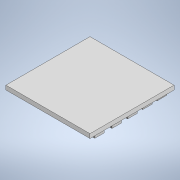
# Autodesk Inventor part: hall_toll
Saved by Autodesk Inventor 2021 (Build 250183000, 183)
## iProperties
Created: 2021-03-01
Part Number: hall_toll
Material: Generic
Document SubType Name: Modeling
Designer: Patrick
Density: 1 g/cm^3
Appearance: Default
Author: Patrick
Autodesk Inventor part; units mm, degrees
(part 1 of 2)
ref_plane "YZ Plane" through (0, 0, 0) normal (1, 0, 0) x (0, 1, 0)
ref_plane "XZ Plane" through (0, 0, 0) normal (0, 1, 0) x (-1, 0, 0)
ref_plane "XY Plane" through (0, 0, 0) normal (0, 0, 1) x (1, 0, 0)
sketch "Sketch1" plane through (0, 0, 0) normal (0, 1, 0) x (-1, 0, 0)
  line L0 (0, -5.8586) -> (50.8, -5.8586)
  line L1 (50.8, -5.8586) -> (50.8, -56.6586)
  line L2 (50.8, -56.6586) -> (0, -56.6586)
  line L3 (0, -56.6586) -> (0, -5.8586)
  line L4 (0, 0) -> (0, 2.7804) construction
  line L5 (15.8266, -10.75) -> (12.7532, -10.75)
  line L6 (12.7532, -10.75) -> (12.7532, -14.7378)
  line L7 (12.7532, -14.7378) -> (15.8266, -14.7378)
  line L8 (15.8266, -14.7378) -> (15.8266, -10.75)
  line L9 (15.8266, -10.75) -> (12.7532, -14.7378) construction
  line L10 (12.7532, -10.75) -> (15.8266, -14.7378) construction
  line L11 (16.6394, -9.9372) -> (11.9404, -9.9372)
  line L12 (11.9404, -9.9372) -> (11.9404, -15.5506)
  line L13 (11.9404, -15.5506) -> (16.6394, -15.5506)
  line L14 (16.6394, -15.5506) -> (16.6394, -9.9372)
  line L15 (16.6394, -9.9372) -> (11.9404, -15.5506) construction
  line L16 (11.9404, -9.9372) -> (16.6394, -15.5506) construction
  line L17 (11.9404, -10.9532) -> (16.6394, -10.9532)
  line L18 (16.6394, -10.9532) -> (16.6394, -14.5346)
  line L19 (16.6394, -14.5346) -> (11.9404, -14.5346)
  line L20 (11.9404, -14.5346) -> (11.9404, -10.9532)
  line L21 (11.9404, -10.9532) -> (16.6394, -14.5346) construction
  line L22 (16.6394, -10.9532) -> (11.9404, -14.5346) construction
  line L23 (15.8118, -21.1328) -> (12.6884, -21.1328)
  line L24 (12.6884, -21.1328) -> (12.6884, -25.1706)
  line L25 (12.6884, -25.1706) -> (15.8118, -25.1706)
  line L26 (15.8118, -25.1706) -> (15.8118, -21.1328)
  line L27 (15.8118, -21.1328) -> (12.6884, -25.1706) construction
  line L28 (12.6884, -21.1328) -> (15.8118, -25.1706) construction
  line L29 (16.6246, -20.32) -> (11.8756, -20.32)
  line L30 (11.8756, -20.32) -> (11.8756, -25.9834)
  line L31 (11.8756, -25.9834) -> (16.6246, -25.9834)
  line L32 (16.6246, -25.9834) -> (16.6246, -20.32)
  line L33 (16.6246, -20.32) -> (11.8756, -25.9834) construction
  line L34 (11.8756, -20.32) -> (16.6246, -25.9834) construction
  line L35 (11.8756, -21.361) -> (16.6246, -21.361)
  line L36 (16.6246, -21.361) -> (16.6246, -24.9424)
  line L37 (16.6246, -24.9424) -> (11.8756, -24.9424)
  line L38 (11.8756, -24.9424) -> (11.8756, -21.361)
  line L39 (11.8756, -21.361) -> (16.6246, -24.9424) construction
  line L40 (16.6246, -21.361) -> (11.8756, -24.9424) construction
  line L41 (12.6374, -34.9027) -> (15.8108, -34.9027)
  line L42 (11.8246, -34.6495) -> (11.8246, -31.0681)
  line L43 (16.6236, -34.6495) -> (11.8246, -34.6495)
  line L44 (11.8246, -35.7155) -> (16.6236, -35.7155)
  line L45 (12.6374, -30.8149) -> (12.6374, -34.9027)
  line L46 (11.8246, -30.0021) -> (11.8246, -35.7155)
  line L47 (15.8108, -30.8149) -> (12.6374, -34.9027) construction
  line L48 (15.8108, -34.9027) -> (15.8108, -30.8149)
  line L49 (12.6374, -30.8149) -> (15.8108, -34.9027) construction
  line L50 (16.6236, -31.0681) -> (11.8246, -34.6495) construction
  line L51 (16.6236, -31.0681) -> (16.6236, -34.6495)
  line L52 (11.8246, -31.0681) -> (16.6236, -34.6495) construction
  line L53 (11.8246, -30.0021) -> (16.6236, -35.7155) construction
  line L54 (16.6236, -30.0021) -> (11.8246, -35.7155) construction
  line L55 (16.6236, -35.7155) -> (16.6236, -30.0021)
  line L56 (11.8246, -31.0681) -> (16.6236, -31.0681)
  line L57 (16.6236, -30.0021) -> (11.8246, -30.0021)
  line L58 (15.8108, -30.8149) -> (12.6374, -30.8149)
  line L59 (15.8942, -40.2355) -> (12.6708, -40.2355)
  line L60 (12.6708, -44.3733) -> (15.8942, -44.3733)
  line L61 (16.707, -40.5137) -> (16.707, -44.0951)
  line L62 (11.858, -44.0951) -> (11.858, -40.5137)
  line L63 (12.6708, -40.2355) -> (12.6708, -44.3733)
  line L64 (15.8942, -44.3733) -> (15.8942, -40.2355)
  line L65 (11.858, -40.5137) -> (16.707, -40.5137)
  line L66 (16.707, -44.0951) -> (11.858, -44.0951)
  line L67 (15.8942, -40.2355) -> (12.6708, -44.3733) construction
  line L68 (12.6708, -40.2355) -> (15.8942, -44.3733) construction
  line L69 (16.707, -39.4227) -> (11.858, -39.4227)
  line L70 (11.858, -45.1861) -> (16.707, -45.1861)
  line L71 (16.707, -40.5137) -> (11.858, -44.0951) construction
  line L72 (11.858, -40.5137) -> (16.707, -44.0951) construction
  line L73 (16.707, -45.1861) -> (16.707, -39.4227)
  line L74 (11.858, -39.4227) -> (16.707, -45.1861) construction
  line L75 (16.707, -39.4227) -> (11.858, -45.1861) construction
  line L76 (11.858, -39.4227) -> (11.858, -45.1861)
  line L77 (12.6807, -53.397) -> (15.9541, -53.397)
  line L78 (11.8679, -53.0938) -> (11.8679, -49.5124)
  line L79 (12.6807, -49.2092) -> (12.6807, -53.397)
  line L80 (16.7669, -53.0938) -> (11.8679, -53.0938)
  line L81 (11.8679, -54.2098) -> (16.7669, -54.2098)
  line L82 (15.9541, -49.2092) -> (12.6807, -53.397) construction
  line L83 (15.9541, -53.397) -> (15.9541, -49.2092)
  line L84 (15.9541, -49.2092) -> (12.6807, -49.2092)
  line L85 (16.7669, -49.5124) -> (16.7669, -53.0938)
  line L86 (11.8679, -48.3964) -> (11.8679, -54.2098)
  line L87 (16.7669, -49.5124) -> (11.8679, -53.0938) construction
  line L88 (11.8679, -49.5124) -> (16.7669, -53.0938) construction
  line L89 (11.8679, -49.5124) -> (16.7669, -49.5124)
  line L90 (16.7669, -48.3964) -> (11.8679, -48.3964)
  line L91 (16.7669, -48.3964) -> (11.8679, -54.2098) construction
  line L92 (11.8679, -48.3964) -> (16.7669, -54.2098) construction
  line L93 (16.7669, -54.2098) -> (16.7669, -48.3964)
  line L94 (12.6807, -49.2092) -> (15.9541, -53.397) construction
  point P0 (14.2899, -12.7439)
  point P1 (14.2899, -12.7439)
  point P2 (14.2899, -12.7439)
  point P3 (14.2899, -12.7439)
  point P4 (14.2899, -12.7439)
  point P5 (14.2501, -23.1517)
  point P6 (14.2501, -23.1517)
  point P7 (14.2501, -23.1517)
  point P8 (14.2501, -23.1517)
  point P9 (14.2501, -23.1517)
  point P10 (14.2241, -32.8588)
  point P11 (14.2241, -32.8588)
  point P12 (14.2241, -32.8588)
  point P13 (14.2241, -32.8588)
  point P14 (14.2241, -32.8588)
  point P15 (14.2825, -42.3044)
  point P16 (14.2825, -42.3044)
  point P17 (14.2825, -42.3044)
  point P18 (14.2825, -42.3044)
  point P19 (14.2825, -42.3044)
  point P20 (14.3174, -51.3031)
  point P21 (14.3174, -51.3031)
  point P22 (14.3174, -51.3031)
  point P23 (14.3174, -51.3031)
  point P24 (14.3174, -51.3031)
  point P25 (12.6807, -53.0938)
  point P26 (12.6807, -49.5124)
  point P27 (12.6708, -44.0951)
  point P28 (12.6708, -40.5137)
  point P29 (12.6374, -34.6495)
  point P30 (12.6374, -31.0681)
  point P31 (12.6884, -21.361)
  point P32 (12.6884, -24.9424)
  point P33 (12.7532, -14.5346)
  point P34 (12.7532, -10.9532)
  dimension "d1" = 50.8
  dimension "d8" = 3.9878
  dimension "d9" = 3.0734
  dimension "d10" = 0.8128
  dimension "d11" = 0.8128
  dimension "d12" = 3.5814
  dimension "d13" = 4.0378
  dimension "d14" = 3.1234
  dimension "d15" = 0.8128
  dimension "d16" = 0.8128
  dimension "d17" = 3.5814
  dimension "d18" = 4.0878
  dimension "d19" = 3.1734
  dimension "d20" = 0.8128
  dimension "d21" = 0.8128
  dimension "d22" = 3.5814
  dimension "d23" = 4.1378
  dimension "d24" = 3.2234
  dimension "d25" = 0.8128
  dimension "d26" = 0.8128
  dimension "d27" = 3.5814
  dimension "d28" = 4.1878
  dimension "d29" = 3.2734
  dimension "d30" = 0.8128
  dimension "d31" = 0.8128
  dimension "d32" = 3.5814
  constraints: 190 end point, 50 midpoint, 32 parallel, 16 horizontal, 16 perpendicular, 5 collinear, 1 vertical
  measures "d1" distance between parallel lines of L3 L1
  measures "d8" distance of L5.end L6.end
  measures "d9" distance between parallel lines of L6 L8
  measures "d10" distance between parallel lines of L13 L7
  measures "d11" distance between parallel lines of L12 L6
  measures "d12" distance between parallel lines of L19 L17
  measures "d13" distance of L24.start L25.start
  measures "d14" distance between parallel lines of L24 L26
  measures "d15" distance between parallel lines of L31 L25
  measures "d16" distance between parallel lines of L30 L24
  measures "d17" distance between parallel lines of L37 L35
  measures "d18" distance of L58.end L41.start
  measures "d19" distance between parallel lines of L45 L48
  measures "d20" distance between parallel lines of L44 L41
  measures "d21" distance between parallel lines of L46 L45
  measures "d22" distance between parallel lines of L43 L56
  measures "d23" distance of L63.start L60.start
  measures "d24" distance between parallel lines of L63 L64
  measures "d25" distance between parallel lines of L70 L60
  measures "d26" distance between parallel lines of L76 L63
  measures "d27" distance between parallel lines of L66 L65
  measures "d28" distance of L84.end L79.end
  measures "d29" distance between parallel lines of L79 L83
  measures "d30" distance between parallel lines of L81 L77
  measures "d31" distance between parallel lines of L86 L79
  measures "d32" distance between parallel lines of L80 L89
extrude "Extrusion2" add sketch "Sketch1" along normal blind 2.54 contours L0 L1 L2 L3 | L8 L17 L6 L5 | L5 L6 L17 L12 L11 L14 L8 | L17 L14 L19 L8 | L8 L19 L6 L17 | L6 L19 L12 L17 | L19 L14 L13 L12 L6 L7 L8 | L8 L7 L6 L19 | L26 L35 L24 L23 | L23 L24 L35 L30 L29 L32 L26 | L35 L32 L37 L26 | L26 L37 L24 L35 | L24 L37 L30 L35 | L37 L32 L31 L30 L24 L25 L26 | L26 L25 L24 L37 | L45 L43 L48 L41 | L41 L48 L43 L55 L44 L46 L45 | L45 L56 L48 L43 | L43 L42 L56 L45 | L48 L56 L51 L43 | L56 L46 L57 L55 L48 L58 L45 | L45 L58 L48 L56 | L64 L65 L63 L59 | L59 L63 L65 L76 L69 L73 L64 | L65 L61 L66 L64 | L64 L66 L63 L65 | L63 L66 L62 L65 | L66 L73 L70 L76 L63 L60 L64 | L64 L60 L63 L66 | L79 L80 L83 L77 | L77 L83 L80 L93 L81 L86 L79 | L80 L78 L89 L79 | L79 L89 L83 L80 | L83 L89 L85 L80 | L89 L86 L90 L93 L83 L84 L79 | L79 L84 L83 L89
sketch "Sketch2" plane through (0, 0, 0) normal (0, -1, 0) x (1, 0, 0)
  line L0 (0, -5.8586) -> (0, -56.6586) projected
  line L1 (-50.8, -5.8586) -> (0, -5.8586) projected
  line L2 (0, -56.6586) -> (-50.8, -56.6586) projected
  line L3 (0, -5.8586) -> (0, -56.6586) projected
  line L4 (-50.8, -5.8586) -> (0, -5.8586) projected
  line L5 (-50.8, -56.6586) -> (-50.8, -5.8586) projected
  line L6 (-2.0206, -10.75) -> (-5.094, -10.75)
  line L7 (-5.094, -10.75) -> (-5.094, -14.7378)
  line L8 (-5.094, -14.7378) -> (-2.0206, -14.7378)
  line L9 (-2.0206, -14.7378) -> (-2.0206, -10.75)
  line L10 (-2.0206, -10.75) -> (-5.094, -14.7378) construction
  line L11 (-5.094, -10.75) -> (-2.0206, -14.7378) construction
  line L12 (-1.2078, -9.9372) -> (-5.9068, -9.9372)
  line L13 (-5.9068, -9.9372) -> (-5.9068, -15.5506)
  line L14 (-5.9068, -15.5506) -> (-1.2078, -15.5506)
  line L15 (-1.2078, -15.5506) -> (-1.2078, -9.9372)
  line L16 (-1.2078, -9.9372) -> (-5.9068, -15.5506) construction
  line L17 (-5.9068, -9.9372) -> (-1.2078, -15.5506) construction
  line L18 (-5.9068, -10.9532) -> (-1.2078, -10.9532)
  line L19 (-1.2078, -10.9532) -> (-1.2078, -14.5346)
  line L20 (-1.2078, -14.5346) -> (-5.9068, -14.5346)
  line L21 (-5.9068, -14.5346) -> (-5.9068, -10.9532)
  line L22 (-5.9068, -10.9532) -> (-1.2078, -14.5346) construction
  line L23 (-1.2078, -10.9532) -> (-5.9068, -14.5346) construction
  line L24 (-5.1065, -25.1706) -> (-1.9831, -25.1706)
  line L25 (-5.9193, -24.9424) -> (-5.9193, -21.361)
  line L26 (-1.1703, -24.9424) -> (-5.9193, -24.9424)
  line L27 (-5.9193, -25.9834) -> (-1.1703, -25.9834)
  line L28 (-5.1065, -21.1328) -> (-5.1065, -25.1706)
  line L29 (-5.9193, -20.32) -> (-5.9193, -25.9834)
  line L30 (-1.9831, -21.1328) -> (-5.1065, -25.1706) construction
  line L31 (-1.9831, -25.1706) -> (-1.9831, -21.1328)
  line L32 (-5.1065, -21.1328) -> (-1.9831, -25.1706) construction
  line L33 (-1.1703, -21.361) -> (-5.9193, -24.9424) construction
  line L34 (-1.1703, -21.361) -> (-1.1703, -24.9424)
  line L35 (-5.9193, -21.361) -> (-1.1703, -24.9424) construction
  line L36 (-5.9193, -20.32) -> (-1.1703, -25.9834) construction
  line L37 (-1.1703, -20.32) -> (-5.9193, -25.9834) construction
  line L38 (-1.1703, -25.9834) -> (-1.1703, -20.32)
  line L39 (-5.9193, -21.361) -> (-1.1703, -21.361)
  line L40 (-1.1703, -20.32) -> (-5.9193, -20.32)
  line L41 (-1.9831, -21.1328) -> (-5.1065, -21.1328)
  line L42 (-2.2323, -30.8149) -> (-5.4057, -30.8149)
  line L43 (-5.4057, -34.9027) -> (-2.2323, -34.9027)
  line L44 (-1.4195, -31.0681) -> (-1.4195, -34.6495)
  line L45 (-6.2185, -34.6495) -> (-6.2185, -31.0681)
  line L46 (-5.4057, -30.8149) -> (-5.4057, -34.9027)
  line L47 (-2.2323, -34.9027) -> (-2.2323, -30.8149)
  line L48 (-6.2185, -31.0681) -> (-1.4195, -31.0681)
  line L49 (-1.4195, -34.6495) -> (-6.2185, -34.6495)
  line L50 (-2.2323, -30.8149) -> (-5.4057, -34.9027) construction
  line L51 (-5.4057, -30.8149) -> (-2.2323, -34.9027) construction
  line L52 (-1.4195, -30.0021) -> (-6.2185, -30.0021)
  line L53 (-6.2185, -35.7155) -> (-1.4195, -35.7155)
  line L54 (-1.4195, -31.0681) -> (-6.2185, -34.6495) construction
  line L55 (-6.2185, -31.0681) -> (-1.4195, -34.6495) construction
  line L56 (-1.4195, -35.7155) -> (-1.4195, -30.0021)
  line L57 (-6.2185, -30.0021) -> (-1.4195, -35.7155) construction
  line L58 (-1.4195, -30.0021) -> (-6.2185, -35.7155) construction
  line L59 (-6.2185, -30.0021) -> (-6.2185, -35.7155)
  line L60 (-5.7968, -44.3733) -> (-2.5734, -44.3733)
  line L61 (-6.6096, -44.0951) -> (-6.6096, -40.5137)
  line L62 (-5.7968, -40.2355) -> (-5.7968, -44.3733)
  line L63 (-1.7606, -44.0951) -> (-6.6096, -44.0951)
  line L64 (-6.6096, -45.1861) -> (-1.7606, -45.1861)
  line L65 (-2.5734, -40.2355) -> (-5.7968, -44.3733) construction
  line L66 (-2.5734, -44.3733) -> (-2.5734, -40.2355)
  line L67 (-2.5734, -40.2355) -> (-5.7968, -40.2355)
  line L68 (-1.7606, -40.5137) -> (-1.7606, -44.0951)
  line L69 (-6.6096, -39.4227) -> (-6.6096, -45.1861)
  line L70 (-1.7606, -40.5137) -> (-6.6096, -44.0951) construction
  line L71 (-6.6096, -40.5137) -> (-1.7606, -44.0951) construction
  line L72 (-6.6096, -40.5137) -> (-1.7606, -40.5137)
  line L73 (-1.7606, -39.4227) -> (-6.6096, -39.4227)
  line L74 (-1.7606, -39.4227) -> (-6.6096, -45.1861) construction
  line L75 (-6.6096, -39.4227) -> (-1.7606, -45.1861) construction
  line L76 (-1.7606, -45.1861) -> (-1.7606, -39.4227)
  line L77 (-5.7968, -40.2355) -> (-2.5734, -44.3733) construction
  line L78 (-2.7966, -49.2092) -> (-6.07, -49.2092)
  line L79 (-6.8828, -53.0938) -> (-6.8828, -49.5124)
  line L80 (-6.8828, -49.5124) -> (-1.9838, -49.5124)
  line L81 (-1.9838, -48.3964) -> (-6.8828, -48.3964)
  line L82 (-6.07, -49.2092) -> (-6.07, -53.397)
  line L83 (-6.8828, -48.3964) -> (-6.8828, -54.2098)
  line L84 (-2.7966, -53.397) -> (-2.7966, -49.2092)
  line L85 (-2.7966, -49.2092) -> (-6.07, -53.397) construction
  line L86 (-6.07, -49.2092) -> (-2.7966, -53.397) construction
  line L87 (-1.9838, -54.2098) -> (-1.9838, -48.3964)
  line L88 (-6.8828, -48.3964) -> (-1.9838, -54.2098) construction
  line L89 (-1.9838, -48.3964) -> (-6.8828, -54.2098) construction
  line L90 (-1.9838, -49.5124) -> (-1.9838, -53.0938)
  line L91 (-1.9838, -49.5124) -> (-6.8828, -53.0938) construction
  line L92 (-6.8828, -49.5124) -> (-1.9838, -53.0938) construction
  line L93 (-6.07, -53.397) -> (-2.7966, -53.397)
  line L94 (-1.9838, -53.0938) -> (-6.8828, -53.0938)
  line L95 (-6.8828, -54.2098) -> (-1.9838, -54.2098)
  point P0 (0, 0)
  point P1 (-3.5573, -12.7439)
  point P2 (-3.5573, -12.7439)
  point P3 (-3.5573, -12.7439)
  point P4 (-3.5573, -12.7439)
  point P5 (-3.5573, -12.7439)
  point P6 (-3.5448, -23.1517)
  point P7 (-3.5448, -23.1517)
  point P8 (-3.5448, -23.1517)
  point P9 (-3.5448, -23.1517)
  point P10 (-3.5448, -23.1517)
  point P11 (-3.819, -32.8588)
  point P12 (-3.819, -32.8588)
  point P13 (-3.819, -32.8588)
  point P14 (-3.819, -32.8588)
  point P15 (-3.819, -32.8588)
  point P16 (-4.1851, -42.3044)
  point P17 (-4.1851, -42.3044)
  point P18 (-4.1851, -42.3044)
  point P19 (-4.1851, -42.3044)
  point P20 (-4.1851, -42.3044)
  point P21 (-4.4333, -51.3031)
  point P22 (-4.4333, -51.3031)
  point P23 (-4.4333, -51.3031)
  point P24 (-4.4333, -51.3031)
  point P25 (-4.4333, -51.3031)
  point P26 (-6.07, -53.0938)
  point P27 (-6.07, -49.5124)
  point P28 (-5.7968, -44.0951)
  point P29 (-5.7968, -40.5137)
  point P30 (-5.4057, -34.6495)
  point P31 (-5.4057, -31.0681)
  point P32 (-5.1065, -24.9424)
  point P33 (-5.1065, -21.361)
  point P34 (-1.2078, -10.9532)
  point P35 (-5.094, -10.9532)
  point P36 (-5.094, -14.5346)
  dimension "d42" = 3.9878
  dimension "d43" = 3.0734
  dimension "d44" = 0.8128
  dimension "d45" = 0.8128
  dimension "d46" = 3.5814
  dimension "d47" = 4.0378
  dimension "d48" = 3.1234
  dimension "d49" = 0.8128
  dimension "d50" = 0.8128
  dimension "d51" = 3.5814
  dimension "d52" = 4.0878
  dimension "d53" = 3.1734
  dimension "d54" = 0.8128
  dimension "d55" = 0.8128
  dimension "d56" = 3.5814
  dimension "d57" = 4.1378
  dimension "d58" = 3.2234
  dimension "d59" = 0.8128
  dimension "d60" = 0.8128
  dimension "d61" = 3.5814
  dimension "d62" = 4.1878
  dimension "d63" = 3.2734
  dimension "d64" = 0.8128
  dimension "d65" = 0.8128
  dimension "d66" = 3.5814
  constraints: 180 end point, 50 midpoint, 31 parallel, 15 horizontal, 15 perpendicular, 5 collinear
  measures "d42" distance of L6.end L7.end
  measures "d43" distance between parallel lines of L7 L9
  measures "d44" distance between parallel lines of L14 L8
  measures "d45" distance between parallel lines of L13 L7
  measures "d46" distance between parallel lines of L20 L18
  measures "d47" distance of L41.end L28.end
  measures "d48" distance between parallel lines of L28 L31
  measures "d49" distance between parallel lines of L27 L24
  measures "d50" distance between parallel lines of L29 L28
  measures "d51" distance between parallel lines of L26 L39
  measures "d52" distance of L42.end L43.start
  measures "d53" distance between parallel lines of L46 L47
  measures "d54" distance between parallel lines of L53 L43
  measures "d55" distance between parallel lines of L59 L46
  measures "d56" distance between parallel lines of L49 L48
  measures "d57" distance of L62.start L60.start
  measures "d58" distance between parallel lines of L62 L66
  measures "d59" distance between parallel lines of L64 L60
  measures "d60" distance between parallel lines of L69 L62
  measures "d61" distance between parallel lines of L63 L72
  measures "d62" distance of L82.start L93.start
  measures "d63" distance between parallel lines of L82 L84
  measures "d64" distance between parallel lines of L95 L93
  measures "d65" distance between parallel lines of L83 L82
  measures "d66" distance between parallel lines of L94 L80
extrude "Extrusion3" add sketch "Sketch2" along normal blind 2.54 contours L6 L7 L18 L13 L12 L15 L9 | L18 L15 L20 L9 | L20 L15 L14 L13 L7 L8 L9 | L24 L31 L26 L38 L27 L29 L28 | L31 L39 L34 L26 | L39 L29 L40 L38 L31 L41 L28 | L42 L46 L48 L59 L52 L56 L47 | L48 L44 L49 L47 | L49 L56 L53 L59 L46 L43 L47 | L60 L66 L63 L76 L64 L69 L62 | L66 L72 L68 L63 | L72 L69 L73 L76 L66 L67 L62 | L78 L82 L80 L83 L81 L87 L84 | L80 L87 L94 L84 | L94 L87 L95 L83 L82 L93 L84
sketch "Sketch3" plane through (0, 0, 0) normal (0, -1, 0) x (1, 0, 0)
  line L0 (-17.2686, -53.397) -> (-13.9952, -53.397)
  line L1 (-18.0814, -53.0938) -> (-18.0814, -49.5124)
  line L2 (-17.2686, -49.2092) -> (-17.2686, -53.397)
  line L3 (-18.0814, -54.2098) -> (-13.1824, -54.2098)
  line L4 (-13.1824, -53.0938) -> (-18.0814, -53.0938)
  line L5 (-18.0814, -48.3964) -> (-18.0814, -54.2098)
  line L6 (-17.2686, -49.2092) -> (-13.9952, -53.397) construction
  line L7 (-13.9952, -49.2092) -> (-17.2686, -49.2092)
  line L8 (-13.9952, -53.397) -> (-13.9952, -49.2092)
  line L9 (-13.9952, -49.2092) -> (-17.2686, -53.397) construction
  line L10 (-13.1824, -49.5124) -> (-18.0814, -53.0938) construction
  line L11 (-18.0814, -49.5124) -> (-13.1824, -53.0938) construction
  line L12 (-13.1824, -48.3964) -> (-18.0814, -54.2098) construction
  line L13 (-18.0814, -48.3964) -> (-13.1824, -54.2098) construction
  line L14 (-13.1824, -48.3964) -> (-18.0814, -48.3964)
  line L15 (-13.1824, -49.5124) -> (-13.1824, -53.0938)
  line L16 (-13.1824, -54.2098) -> (-13.1824, -48.3964)
  line L17 (-13.8564, -10.75) -> (-16.9298, -10.75)
  line L18 (-17.7426, -14.5346) -> (-17.7426, -10.9532)
  line L19 (-16.9298, -10.75) -> (-16.9298, -14.7378)
  line L20 (-13.0436, -9.9372) -> (-17.7426, -9.9372)
  line L21 (-17.7426, -10.9532) -> (-13.0436, -10.9532)
  line L22 (-17.7426, -9.9372) -> (-17.7426, -15.5506)
  line L23 (-16.9298, -14.7378) -> (-13.8564, -14.7378)
  line L24 (-13.8564, -14.7378) -> (-13.8564, -10.75)
  line L25 (-13.8564, -10.75) -> (-16.9298, -14.7378) construction
  line L26 (-16.9298, -10.75) -> (-13.8564, -14.7378) construction
  line L27 (-13.0436, -14.5346) -> (-17.7426, -14.5346)
  line L28 (-13.0436, -10.9532) -> (-17.7426, -14.5346) construction
  line L29 (-13.0436, -10.9532) -> (-13.0436, -14.5346)
  line L30 (-17.7426, -10.9532) -> (-13.0436, -14.5346) construction
  line L31 (-13.0436, -9.9372) -> (-17.7426, -15.5506) construction
  line L32 (-17.7426, -9.9372) -> (-13.0436, -15.5506) construction
  line L33 (-13.0436, -15.5506) -> (-13.0436, -9.9372)
  line L34 (-14.2485, -21.1328) -> (-17.3719, -21.1328)
  line L35 (-18.1847, -24.9424) -> (-18.1847, -21.361)
  line L36 (-17.3719, -21.1328) -> (-17.3719, -25.1706)
  line L37 (-18.1847, -21.361) -> (-13.4357, -21.361)
  line L38 (-13.4357, -20.32) -> (-18.1847, -20.32)
  line L39 (-17.3719, -25.1706) -> (-14.2485, -25.1706)
  line L40 (-14.2485, -21.1328) -> (-17.3719, -25.1706) construction
  line L41 (-17.3719, -21.1328) -> (-14.2485, -25.1706) construction
  line L42 (-13.4357, -21.361) -> (-13.4357, -24.9424)
  line L43 (-18.1847, -20.32) -> (-18.1847, -25.9834)
  line L44 (-13.4357, -24.9424) -> (-18.1847, -24.9424)
  line L45 (-18.1847, -21.361) -> (-13.4357, -24.9424) construction
  line L46 (-13.4357, -21.361) -> (-18.1847, -24.9424) construction
  line L47 (-18.1847, -25.9834) -> (-13.4357, -25.9834)
  line L48 (-18.1847, -20.32) -> (-13.4357, -25.9834) construction
  line L49 (-13.4357, -20.32) -> (-18.1847, -25.9834) construction
  line L50 (-13.4357, -25.9834) -> (-13.4357, -20.32)
  line L51 (-14.2485, -25.1706) -> (-14.2485, -21.1328)
  line L52 (-17.7426, -15.5506) -> (-13.0436, -15.5506)
  line L53 (-13.86, -31.0681) -> (-13.86, -34.6495)
  line L54 (-14.6728, -30.8149) -> (-17.8462, -30.8149)
  line L55 (-14.6728, -34.9027) -> (-14.6728, -30.8149)
  line L56 (-18.659, -31.0681) -> (-13.86, -31.0681)
  line L57 (-13.86, -30.0021) -> (-18.659, -30.0021)
  line L58 (-17.8462, -34.9027) -> (-14.6728, -34.9027)
  line L59 (-14.6728, -30.8149) -> (-17.8462, -34.9027) construction
  line L60 (-17.8462, -30.8149) -> (-14.6728, -34.9027) construction
  line L61 (-13.86, -35.7155) -> (-13.86, -30.0021)
  line L62 (-13.86, -31.0681) -> (-18.659, -34.6495) construction
  line L63 (-13.86, -34.6495) -> (-18.659, -34.6495)
  line L64 (-18.659, -31.0681) -> (-13.86, -34.6495) construction
  line L65 (-18.659, -35.7155) -> (-13.86, -35.7155)
  line L66 (-13.86, -30.0021) -> (-18.659, -35.7155) construction
  line L67 (-18.659, -30.0021) -> (-13.86, -35.7155) construction
  line L68 (-18.659, -34.6495) -> (-18.659, -31.0681)
  line L69 (-18.659, -30.0021) -> (-18.659, -35.7155)
  line L70 (-17.8462, -30.8149) -> (-17.8462, -34.9027)
  line L71 (-17.9488, -44.3733) -> (-14.7254, -44.3733)
  line L72 (-18.7616, -44.0951) -> (-18.7616, -40.5137)
  line L73 (-13.9126, -44.0951) -> (-18.7616, -44.0951)
  line L74 (-18.7616, -45.1861) -> (-13.9126, -45.1861)
  line L75 (-17.9488, -40.2355) -> (-17.9488, -44.3733)
  line L76 (-18.7616, -39.4227) -> (-18.7616, -45.1861)
  line L77 (-14.7254, -40.2355) -> (-17.9488, -44.3733) construction
  line L78 (-14.7254, -44.3733) -> (-14.7254, -40.2355)
  line L79 (-17.9488, -40.2355) -> (-14.7254, -44.3733) construction
  line L80 (-13.9126, -40.5137) -> (-18.7616, -44.0951) construction
  line L81 (-18.7616, -40.5137) -> (-13.9126, -44.0951) construction
  line L82 (-13.9126, -40.5137) -> (-13.9126, -44.0951)
  line L83 (-13.9126, -39.4227) -> (-18.7616, -45.1861) construction
  line L84 (-18.7616, -39.4227) -> (-13.9126, -45.1861) construction
  line L85 (-13.9126, -45.1861) -> (-13.9126, -39.4227)
  line L86 (-14.7254, -40.2355) -> (-17.9488, -40.2355)
  line L87 (-18.7616, -40.5137) -> (-13.9126, -40.5137)
  line L88 (-13.9126, -39.4227) -> (-18.7616, -39.4227)
  line L89 (-18.0814, -49.5124) -> (-13.1824, -49.5124)
  point P0 (0, 0)
  point P1 (-15.6319, -51.3031)
  point P2 (-15.6319, -51.3031)
  point P3 (-15.6319, -51.3031)
  point P4 (-15.6319, -51.3031)
  point P5 (-15.6319, -51.3031)
  point P6 (-15.3931, -12.7439)
  point P7 (-15.3931, -12.7439)
  point P8 (-15.3931, -12.7439)
  point P9 (-15.3931, -12.7439)
  point P10 (-15.3931, -12.7439)
  point P11 (-15.8102, -23.1517)
  point P12 (-15.8102, -23.1517)
  point P13 (-15.8102, -23.1517)
  point P14 (-15.8102, -23.1517)
  point P15 (-15.8102, -23.1517)
  point P16 (-16.2595, -32.8588)
  point P17 (-16.2595, -32.8588)
  point P18 (-16.2595, -32.8588)
  point P19 (-16.2595, -32.8588)
  point P20 (-16.2595, -32.8588)
  point P21 (-16.3371, -42.3044)
  point P22 (-16.3371, -42.3044)
  point P23 (-16.3371, -42.3044)
  point P24 (-16.3371, -42.3044)
  point P25 (-16.3371, -42.3044)
  point P26 (-13.9952, -49.5124)
  point P27 (-13.9952, -53.0938)
  point P28 (-14.7254, -40.5137)
  point P29 (-14.7254, -44.0951)
  point P30 (-14.6728, -31.0681)
  point P31 (-14.6728, -34.6495)
  point P32 (-14.2485, -24.9424)
  point P33 (-14.2485, -21.361)
  point P34 (-13.8564, -10.9532)
  point P35 (-13.8564, -14.5346)
  dimension "d69" = 3.9878
  dimension "d70" = 3.0734
  dimension "d71" = 0.8128
  dimension "d72" = 0.8128
  dimension "d73" = 3.5814
  dimension "d74" = 4.0378
  dimension "d75" = 3.1234
  dimension "d76" = 0.8128
  dimension "d77" = 0.8128
  dimension "d78" = 3.5814
  dimension "d79" = 4.0878
  dimension "d80" = 3.1734
  dimension "d81" = 0.8128
  dimension "d82" = 0.8128
  dimension "d83" = 3.5814
  dimension "d84" = 4.1378
  dimension "d85" = 3.2234
  dimension "d86" = 0.8128
  dimension "d87" = 0.8128
  dimension "d88" = 3.5814
  dimension "d89" = 4.1878
  dimension "d90" = 3.2734
  dimension "d91" = 0.8128
  dimension "d92" = 0.8128
  dimension "d93" = 3.5814
  constraints: 180 end point, 50 midpoint, 31 parallel, 15 horizontal, 15 perpendicular, 5 collinear
  measures "d69" distance of L17.end L19.end
  measures "d70" distance between parallel lines of L19 L24
  measures "d71" distance between parallel lines of L52 L23
  measures "d72" distance between parallel lines of L22 L19
  measures "d73" distance between parallel lines of L27 L21
  measures "d74" distance of L36.start L39.start
  measures "d75" distance between parallel lines of L36 L51
  measures "d76" distance between parallel lines of L47 L39
  measures "d77" distance between parallel lines of L43 L36
  measures "d78" distance between parallel lines of L44 L37
  measures "d79" distance of L70.start L58.start
  measures "d80" distance between parallel lines of L70 L55
  measures "d81" distance between parallel lines of L65 L58
  measures "d82" distance between parallel lines of L69 L70
  measures "d83" distance between parallel lines of L63 L56
  measures "d84" distance of L86.end L71.start
  measures "d85" distance between parallel lines of L75 L78
  measures "d86" distance between parallel lines of L74 L71
  measures "d87" distance between parallel lines of L76 L75
  measures "d88" distance between parallel lines of L73 L87
  measures "d89" distance of L7.end L2.end
  measures "d90" distance between parallel lines of L2 L8
  measures "d91" distance between parallel lines of L3 L0
  measures "d92" distance between parallel lines of L5 L2
  measures "d93" distance between parallel lines of L4 L89
extrude "Extrusion4" add sketch "Sketch3" along normal blind 2.286 contours L0 L8 L4 L16 L3 L5 L2 | L4 L1 L89 L2 | L89 L5 L14 L16 L8 L7 L2 | L17 L19 L21 L22 L20 L33 L24 | L19 L27 L18 L21 | L27 L33 L52 L22 L19 L23 L24 | L34 L36 L37 L43 L38 L50 L51 | L36 L44 L35 L37 | L44 L50 L47 L43 L36 L39 L51 | L56 L55 L54 L70 L69 L57 L61 | L61 L65 L69 L63 L70 L58 L55 | L70 L63 L68 L56 | L71 L78 L73 L85 L74 L76 L75 | L73 L72 L87 L75 | L87 L76 L88 L85 L78 L86 L75
sketch "Sketch4" plane through (0, 0, 0) normal (0, -1, 0) x (1, 0, 0)
  line L0 (-22.7024, -49.2092) -> (-25.9758, -49.2092)
  line L1 (-27.2218, -45.1861) -> (-22.3728, -45.1861)
  line L2 (-26.2026, -25.1706) -> (-23.0792, -25.1706)
  line L3 (-22.2664, -21.361) -> (-22.2664, -24.9424)
  line L4 (-27.0154, -25.9834) -> (-22.2664, -25.9834)
  line L5 (-22.2664, -24.9424) -> (-27.0154, -24.9424)
  line L6 (-23.0792, -25.1706) -> (-23.0792, -21.1328)
  line L7 (-22.2664, -25.9834) -> (-22.2664, -20.32)
  line L8 (-26.2026, -21.1328) -> (-26.2026, -25.1706)
  line L9 (-23.0792, -21.1328) -> (-26.2026, -25.1706) construction
  line L10 (-26.2026, -21.1328) -> (-23.0792, -25.1706) construction
  line L11 (-27.0154, -21.361) -> (-22.2664, -24.9424) construction
  line L12 (-27.0154, -20.32) -> (-27.0154, -25.9834)
  line L13 (-27.0154, -20.32) -> (-22.2664, -25.9834) construction
  line L14 (-22.2664, -20.32) -> (-27.0154, -25.9834) construction
  line L15 (-27.0154, -24.9424) -> (-27.0154, -21.361)
  line L16 (-22.2664, -21.361) -> (-27.0154, -24.9424) construction
  line L17 (-27.0154, -21.361) -> (-22.2664, -21.361)
  line L18 (-22.2664, -20.32) -> (-27.0154, -20.32)
  line L19 (-23.0792, -21.1328) -> (-26.2026, -21.1328)
  line L20 (-22.6254, -10.75) -> (-25.6988, -10.75)
  line L21 (-26.5116, -14.5346) -> (-26.5116, -10.9532)
  line L22 (-25.6988, -10.75) -> (-25.6988, -14.7378)
  line L23 (-21.8126, -9.9372) -> (-26.5116, -9.9372)
  line L24 (-22.6254, -10.75) -> (-25.6988, -14.7378) construction
  line L25 (-25.6988, -14.7378) -> (-22.6254, -14.7378)
  line L26 (-22.6254, -14.7378) -> (-22.6254, -10.75)
  line L27 (-25.6988, -10.75) -> (-22.6254, -14.7378) construction
  line L28 (-21.8126, -10.9532) -> (-21.8126, -14.5346)
  line L29 (-26.5116, -9.9372) -> (-26.5116, -15.5506)
  line L30 (-21.8126, -14.5346) -> (-26.5116, -14.5346)
  line L31 (-26.5116, -10.9532) -> (-21.8126, -14.5346) construction
  line L32 (-21.8126, -10.9532) -> (-26.5116, -14.5346) construction
  line L33 (-21.8126, -15.5506) -> (-21.8126, -9.9372)
  line L34 (-26.5116, -9.9372) -> (-21.8126, -15.5506) construction
  line L35 (-21.8126, -9.9372) -> (-26.5116, -15.5506) construction
  line L36 (-26.5116, -15.5506) -> (-21.8126, -15.5506)
  line L37 (-26.5116, -10.9532) -> (-21.8126, -10.9532)
  line L38 (-26.6869, -31.0681) -> (-21.8879, -31.0681)
  line L39 (-25.8741, -34.9027) -> (-22.7007, -34.9027)
  line L40 (-21.8879, -34.6495) -> (-26.6869, -34.6495)
  line L41 (-26.6869, -35.7155) -> (-21.8879, -35.7155)
  line L42 (-26.6869, -34.6495) -> (-26.6869, -31.0681)
  line L43 (-25.8741, -30.8149) -> (-25.8741, -34.9027)
  line L44 (-22.7007, -30.8149) -> (-25.8741, -30.8149)
  line L45 (-22.7007, -34.9027) -> (-22.7007, -30.8149)
  line L46 (-25.8741, -30.8149) -> (-22.7007, -34.9027) construction
  line L47 (-22.7007, -30.8149) -> (-25.8741, -34.9027) construction
  line L48 (-21.8879, -31.0681) -> (-26.6869, -34.6495) construction
  line L49 (-26.6869, -31.0681) -> (-21.8879, -34.6495) construction
  line L50 (-26.6869, -30.0021) -> (-26.6869, -35.7155)
  line L51 (-21.8879, -30.0021) -> (-26.6869, -35.7155) construction
  line L52 (-21.8879, -30.0021) -> (-26.6869, -30.0021)
  line L53 (-26.6869, -30.0021) -> (-21.8879, -35.7155) construction
  line L54 (-21.8879, -31.0681) -> (-21.8879, -34.6495)
  line L55 (-21.8879, -35.7155) -> (-21.8879, -30.0021)
  line L56 (-23.1856, -40.2355) -> (-26.409, -40.2355)
  line L57 (-22.3728, -39.4227) -> (-27.2218, -39.4227)
  line L58 (-27.2218, -40.5137) -> (-22.3728, -40.5137)
  line L59 (-27.2218, -44.0951) -> (-27.2218, -40.5137)
  line L60 (-22.3728, -40.5137) -> (-22.3728, -44.0951)
  line L61 (-26.409, -44.3733) -> (-23.1856, -44.3733)
  line L62 (-26.409, -40.2355) -> (-26.409, -44.3733)
  line L63 (-23.1856, -40.2355) -> (-26.409, -44.3733) construction
  line L64 (-23.1856, -44.3733) -> (-23.1856, -40.2355)
  line L65 (-26.409, -40.2355) -> (-23.1856, -44.3733) construction
  line L66 (-22.3728, -44.0951) -> (-27.2218, -44.0951)
  line L67 (-22.3728, -40.5137) -> (-27.2218, -44.0951) construction
  line L68 (-27.2218, -40.5137) -> (-22.3728, -44.0951) construction
  line L69 (-27.2218, -39.4227) -> (-27.2218, -45.1861)
  line L70 (-22.3728, -39.4227) -> (-27.2218, -45.1861) construction
  line L71 (-27.2218, -39.4227) -> (-22.3728, -45.1861) construction
  line L72 (-22.3728, -45.1861) -> (-22.3728, -39.4227)
  line L73 (-26.7886, -49.5124) -> (-21.8896, -49.5124)
  line L74 (-21.8896, -48.3964) -> (-26.7886, -48.3964)
  line L75 (-26.7886, -53.0938) -> (-26.7886, -49.5124)
  line L76 (-25.9758, -49.2092) -> (-25.9758, -53.397)
  line L77 (-25.9758, -53.397) -> (-22.7024, -53.397)
  line L78 (-26.7886, -48.3964) -> (-26.7886, -54.2098)
  line L79 (-25.9758, -49.2092) -> (-22.7024, -53.397) construction
  line L80 (-22.7024, -53.397) -> (-22.7024, -49.2092)
  line L81 (-22.7024, -49.2092) -> (-25.9758, -53.397) construction
  line L82 (-21.8896, -53.0938) -> (-26.7886, -53.0938)
  line L83 (-21.8896, -49.5124) -> (-26.7886, -53.0938) construction
  line L84 (-21.8896, -49.5124) -> (-21.8896, -53.0938)
  line L85 (-26.7886, -54.2098) -> (-21.8896, -54.2098)
  line L86 (-26.7886, -48.3964) -> (-21.8896, -54.2098) construction
  line L87 (-21.8896, -48.3964) -> (-26.7886, -54.2098) construction
  line L88 (-21.8896, -54.2098) -> (-21.8896, -48.3964)
  line L89 (-26.7886, -49.5124) -> (-21.8896, -53.0938) construction
  point P0 (0, 0)
  point P1 (-24.1621, -12.7439)
  point P2 (-24.1621, -12.7439)
  point P3 (-24.6409, -23.1517)
  point P4 (-24.6409, -23.1517)
  point P5 (-24.6409, -23.1517)
  point P6 (-24.6409, -23.1517)
  point P7 (-24.6409, -23.1517)
  point P8 (-24.1621, -12.7439)
  point P9 (-24.1621, -12.7439)
  point P10 (-24.1621, -12.7439)
  point P11 (-24.2874, -32.8588)
  point P12 (-24.2874, -32.8588)
  point P13 (-24.2874, -32.8588)
  point P14 (-24.2874, -32.8588)
  point P15 (-24.2874, -32.8588)
  point P16 (-24.7973, -42.3044)
  point P17 (-24.7973, -42.3044)
  point P18 (-24.7973, -42.3044)
  point P19 (-24.7973, -42.3044)
  point P20 (-24.7973, -42.3044)
  point P21 (-24.3391, -51.3031)
  point P22 (-24.3391, -51.3031)
  point P23 (-24.3391, -51.3031)
  point P24 (-24.3391, -51.3031)
  point P25 (-24.3391, -51.3031)
  point P26 (-25.9758, -53.0938)
  point P27 (-25.9758, -49.5124)
  point P28 (-26.409, -44.0951)
  point P29 (-26.409, -40.5137)
  point P30 (-25.8741, -34.6495)
  point P31 (-25.8741, -31.0681)
  point P32 (-26.2026, -21.361)
  point P33 (-26.2026, -24.9424)
  point P34 (-25.6988, -10.9532)
  point P35 (-25.6988, -14.5346)
  dimension "d96" = 3.9878
  dimension "d97" = 3.0734
  dimension "d98" = 0.8128
  dimension "d99" = 0.8128
  dimension "d100" = 3.5814
  dimension "d101" = 4.0378
  dimension "d102" = 3.1234
  dimension "d103" = 0.8128
  dimension "d104" = 0.8128
  dimension "d105" = 3.5814
  dimension "d106" = 4.0878
  dimension "d107" = 3.1734
  dimension "d108" = 0.8128
  dimension "d109" = 0.8128
  dimension "d110" = 3.5814
  dimension "d111" = 4.1378
  dimension "d112" = 3.2234
  dimension "d113" = 0.8128
  dimension "d114" = 0.8128
  dimension "d115" = 3.5814
  dimension "d116" = 4.1878
  dimension "d117" = 3.2734
  dimension "d118" = 0.8128
  dimension "d119" = 0.8128
  dimension "d120" = 3.5814
  constraints: 180 end point, 50 midpoint, 31 parallel, 15 horizontal, 15 perpendicular, 5 collinear
  measures "d96" distance of L20.end L25.start
  measures "d97" distance between parallel lines of L22 L26
  measures "d98" distance between parallel lines of L36 L25
  measures "d99" distance between parallel lines of L29 L22
  measures "d100" distance between parallel lines of L30 L37
  measures "d101" distance of L8.start L8.end
  measures "d102" distance between parallel lines of L8 L6
  measures "d103" distance between parallel lines of L4 L2
  measures "d104" distance between parallel lines of L12 L8
  measures "d105" distance between parallel lines of L5 L17
  measures "d106" distance of L43.start L39.start
  measures "d107" distance between parallel lines of L43 L45
  measures "d108" distance between parallel lines of L41 L39
  measures "d109" distance between parallel lines of L50 L43
  measures "d110" distance between parallel lines of L40 L38
  measures "d111" distance of L62.start L62.end
  measures "d112" distance between parallel lines of L62 L64
  measures "d113" distance between parallel lines of L1 L61
  measures "d114" distance between parallel lines of L69 L62
  measures "d115" distance between parallel lines of L66 L58
  measures "d116" distance of L76.start L77.start
  measures "d117" distance between parallel lines of L76 L80
  measures "d118" distance between parallel lines of L85 L77
  measures "d119" distance between parallel lines of L78 L76
  measures "d120" distance between parallel lines of L82 L73
extrude "Extrusion5" add sketch "Sketch4" along normal blind 2.032 contours L0 L76 L73 L78 L74 L88 L80 | L73 L84 L82 L80 | L82 L88 L85 L78 L76 L77 L80 | L69 L66 L62 L61 L64 L72 L1 | L66 L64 L58 L60 | L69 L57 L72 L58 L64 L56 L62 | L2 L6 L5 L7 L4 L12 L8 | L6 L17 L3 L5 | L17 L12 L18 L7 L6 L19 L8 | L20 L22 L37 L29 L23 L33 L26 | L37 L28 L30 L26 | L30 L33 L36 L29 L22 L25 L26 | L50 L52 L55 L38 L45 L44 L43 | L40 L43 L39 L45 L55 L41 L50 | L38 L54 L40 L45
sketch "Sketch5" plane through (0, 0, 0) normal (0, -1, 0) x (1, 0, 0)
  line L0 (-37.5662, -45.1861) -> (-32.7172, -45.1861)
  line L1 (-32.7172, -44.0951) -> (-37.5662, -44.0951)
  line L2 (-37.5662, -44.0951) -> (-37.5662, -40.5137)
  line L3 (-36.7534, -40.2355) -> (-36.7534, -44.3733)
  line L4 (-37.5662, -39.4227) -> (-37.5662, -45.1861)
  line L5 (-33.53, -44.3733) -> (-33.53, -40.2355)
  line L6 (-33.53, -40.2355) -> (-36.7534, -40.2355)
  line L7 (-33.53, -40.2355) -> (-36.7534, -44.3733) construction
  line L8 (-36.7534, -40.2355) -> (-33.53, -44.3733) construction
  line L9 (-32.7172, -40.5137) -> (-37.5662, -44.0951) construction
  line L10 (-37.5662, -40.5137) -> (-32.7172, -40.5137)
  line L11 (-37.5662, -40.5137) -> (-32.7172, -44.0951) construction
  line L12 (-32.7172, -45.1861) -> (-32.7172, -39.4227)
  line L13 (-37.5662, -39.4227) -> (-32.7172, -45.1861) construction
  line L14 (-32.7172, -39.4227) -> (-37.5662, -45.1861) construction
  line L15 (-32.7172, -39.4227) -> (-37.5662, -39.4227)
  line L16 (-36.7534, -44.3733) -> (-33.53, -44.3733)
  line L17 (-32.7172, -40.5137) -> (-32.7172, -44.0951)
  line L18 (-37.1253, -21.1328) -> (-37.1253, -25.1706)
  line L19 (-37.9381, -20.32) -> (-37.9381, -25.9834)
  line L20 (-34.0019, -25.1706) -> (-34.0019, -21.1328)
  line L21 (-37.1253, -25.1706) -> (-34.0019, -25.1706)
  line L22 (-34.0019, -21.1328) -> (-37.1253, -25.1706) construction
  line L23 (-37.1253, -21.1328) -> (-34.0019, -25.1706) construction
  line L24 (-37.9381, -21.361) -> (-33.1891, -21.361)
  line L25 (-33.1891, -21.361) -> (-37.9381, -24.9424) construction
  line L26 (-37.9381, -21.361) -> (-33.1891, -24.9424) construction
  line L27 (-33.1891, -24.9424) -> (-37.9381, -24.9424)
  line L28 (-33.1891, -20.32) -> (-37.9381, -20.32)
  line L29 (-37.9381, -25.9834) -> (-33.1891, -25.9834)
  line L30 (-37.9381, -20.32) -> (-33.1891, -25.9834) construction
  line L31 (-33.1891, -20.32) -> (-37.9381, -25.9834) construction
  line L32 (-33.1891, -25.9834) -> (-33.1891, -20.32)
  line L33 (-33.1891, -21.361) -> (-33.1891, -24.9424)
  line L34 (-36.8342, -53.397) -> (-33.5608, -53.397)
  line L35 (-37.647, -53.0938) -> (-37.647, -49.5124)
  line L36 (-37.647, -54.2098) -> (-32.748, -54.2098)
  line L37 (-32.748, -53.0938) -> (-37.647, -53.0938)
  line L38 (-36.8342, -49.2092) -> (-36.8342, -53.397)
  line L39 (-37.647, -48.3964) -> (-37.647, -54.2098)
  line L40 (-33.5608, -49.2092) -> (-36.8342, -53.397) construction
  line L41 (-36.8342, -49.2092) -> (-33.5608, -53.397) construction
  line L42 (-33.5608, -53.397) -> (-33.5608, -49.2092)
  line L43 (-32.748, -49.5124) -> (-37.647, -53.0938) construction
  line L44 (-32.748, -49.5124) -> (-32.748, -53.0938)
  line L45 (-37.647, -49.5124) -> (-32.748, -53.0938) construction
  line L46 (-32.748, -48.3964) -> (-37.647, -54.2098) construction
  line L47 (-32.748, -54.2098) -> (-32.748, -48.3964)
  line L48 (-37.647, -48.3964) -> (-32.748, -54.2098) construction
  line L49 (-33.5608, -49.2092) -> (-36.8342, -49.2092)
  line L50 (-32.748, -48.3964) -> (-37.647, -48.3964)
  line L51 (-37.9381, -24.9424) -> (-37.9381, -21.361)
  line L52 (-32.9923, -10.9532) -> (-32.9923, -14.5346)
  line L53 (-36.8785, -14.7378) -> (-33.8051, -14.7378)
  line L54 (-33.8051, -14.7378) -> (-33.8051, -10.75)
  line L55 (-37.6913, -15.5506) -> (-32.9923, -15.5506)
  line L56 (-33.8051, -10.75) -> (-36.8785, -10.75)
  line L57 (-33.8051, -10.75) -> (-36.8785, -14.7378) construction
  line L58 (-36.8785, -10.75) -> (-36.8785, -14.7378)
  line L59 (-36.8785, -10.75) -> (-33.8051, -14.7378) construction
  line L60 (-32.9923, -15.5506) -> (-32.9923, -9.9372)
  line L61 (-32.9923, -10.9532) -> (-37.6913, -14.5346) construction
  line L62 (-37.6913, -10.9532) -> (-32.9923, -10.9532)
  line L63 (-37.6913, -14.5346) -> (-37.6913, -10.9532)
  line L64 (-37.6913, -10.9532) -> (-32.9923, -14.5346) construction
  line L65 (-32.9923, -9.9372) -> (-37.6913, -9.9372)
  line L66 (-37.6913, -9.9372) -> (-37.6913, -15.5506)
  line L67 (-37.6913, -9.9372) -> (-32.9923, -15.5506) construction
  line L68 (-32.9923, -9.9372) -> (-37.6913, -15.5506) construction
  line L69 (-32.9923, -14.5346) -> (-37.6913, -14.5346)
  line L70 (-37.0538, -34.9027) -> (-33.8804, -34.9027)
  line L71 (-37.8666, -34.6495) -> (-37.8666, -31.0681)
  line L72 (-37.8666, -35.7155) -> (-33.0676, -35.7155)
  line L73 (-33.0676, -34.6495) -> (-37.8666, -34.6495)
  line L74 (-37.0538, -30.8149) -> (-37.0538, -34.9027)
  line L75 (-37.8666, -30.0021) -> (-37.8666, -35.7155)
  line L76 (-33.8804, -30.8149) -> (-37.0538, -30.8149)
  line L77 (-33.8804, -30.8149) -> (-37.0538, -34.9027) construction
  line L78 (-37.0538, -30.8149) -> (-33.8804, -34.9027) construction
  line L79 (-33.0676, -31.0681) -> (-37.8666, -34.6495) construction
  line L80 (-37.8666, -31.0681) -> (-33.0676, -31.0681)
  line L81 (-37.8666, -31.0681) -> (-33.0676, -34.6495) construction
  line L82 (-33.0676, -30.0021) -> (-37.8666, -35.7155) construction
  line L83 (-33.0676, -30.0021) -> (-37.8666, -30.0021)
  line L84 (-37.8666, -30.0021) -> (-33.0676, -35.7155) construction
  line L85 (-33.0676, -35.7155) -> (-33.0676, -30.0021)
  line L86 (-33.0676, -31.0681) -> (-33.0676, -34.6495)
  line L87 (-33.8804, -34.9027) -> (-33.8804, -30.8149)
  line L88 (-34.0019, -21.1328) -> (-37.1253, -21.1328)
  line L89 (-37.647, -49.5124) -> (-32.748, -49.5124)
  point P0 (0, 0)
  point P1 (-35.1417, -42.3044)
  point P2 (-35.1417, -42.3044)
  point P3 (-35.1417, -42.3044)
  point P4 (-35.1417, -42.3044)
  point P5 (-35.1417, -42.3044)
  point P6 (-35.5636, -23.1517)
  point P7 (-35.5636, -23.1517)
  point P8 (-35.5636, -23.1517)
  point P9 (-35.5636, -23.1517)
  point P10 (-35.5636, -23.1517)
  point P11 (-35.1975, -51.3031)
  point P12 (-35.1975, -51.3031)
  point P13 (-35.1975, -51.3031)
  point P14 (-35.1975, -51.3031)
  point P15 (-35.1975, -51.3031)
  point P16 (-35.3418, -12.7439)
  point P17 (-35.3418, -12.7439)
  point P18 (-35.3418, -12.7439)
  point P19 (-35.3418, -12.7439)
  point P20 (-35.3418, -12.7439)
  point P21 (-35.4671, -32.8588)
  point P22 (-35.4671, -32.8588)
  point P23 (-35.4671, -32.8588)
  point P24 (-35.4671, -32.8588)
  point P25 (-35.4671, -32.8588)
  point P26 (-33.5608, -49.5124)
  point P27 (-33.5608, -53.0938)
  point P28 (-33.53, -40.5137)
  point P29 (-33.53, -44.0951)
  point P30 (-33.8804, -31.0681)
  point P31 (-33.8804, -34.6495)
  point P32 (-34.0019, -21.361)
  point P33 (-34.0019, -24.9424)
  point P34 (-33.8051, -10.9532)
  point P35 (-33.8051, -14.5346)
  dimension "d123" = 3.9878
  dimension "d124" = 3.0734
  dimension "d125" = 0.8128
  dimension "d126" = 0.8128
  dimension "d127" = 3.5814
  dimension "d128" = 4.0378
  dimension "d129" = 3.1234
  dimension "d130" = 0.8128
  dimension "d131" = 0.8128
  dimension "d132" = 3.5814
  dimension "d133" = 4.0878
  dimension "d134" = 3.1734
  dimension "d135" = 0.8128
  dimension "d136" = 0.8128
  dimension "d137" = 3.5814
  dimension "d138" = 4.1378
  dimension "d139" = 3.2234
  dimension "d140" = 0.8128
  dimension "d141" = 0.8128
  dimension "d142" = 3.5814
  dimension "d143" = 4.1878
  dimension "d144" = 3.2734
  dimension "d145" = 0.8128
  dimension "d146" = 0.8128
  dimension "d147" = 3.5814
  constraints: 180 end point, 50 midpoint, 31 parallel, 15 horizontal, 15 perpendicular, 5 collinear
  measures "d123" distance of L56.end L58.end
  measures "d124" distance between parallel lines of L58 L54
  measures "d125" distance between parallel lines of L55 L53
  measures "d126" distance between parallel lines of L66 L58
  measures "d127" distance between parallel lines of L69 L62
  measures "d128" distance of L18.start L21.start
  measures "d129" distance between parallel lines of L18 L20
  measures "d130" distance between parallel lines of L29 L21
  measures "d131" distance between parallel lines of L19 L18
  measures "d132" distance between parallel lines of L27 L24
  measures "d133" distance of L74.start L70.start
  measures "d134" distance between parallel lines of L74 L87
  measures "d135" distance between parallel lines of L72 L70
  measures "d136" distance between parallel lines of L75 L74
  measures "d137" distance between parallel lines of L73 L80
  measures "d138" distance of L3.start L3.end
  measures "d139" distance between parallel lines of L3 L5
  measures "d140" distance between parallel lines of L0 L16
  measures "d141" distance between parallel lines of L4 L3
  measures "d142" distance between parallel lines of L1 L10
  measures "d143" distance of L38.start L34.start
  measures "d144" distance between parallel lines of L38 L42
  measures "d145" distance between parallel lines of L36 L34
  measures "d146" distance between parallel lines of L39 L38
  measures "d147" distance between parallel lines of L37 L89
extrude "Extrusion6" add sketch "Sketch5" along normal blind 1.778 contours L4 L1 L3 L16 L5 L12 L0 | L2 L10 L3 L1 | L4 L15 L12 L10 L5 L6 L3 | L18 L24 L19 L28 L32 L20 L88 | L18 L27 L19 L24 | L18 L21 L20 L27 L32 L29 L19 | L34 L42 L37 L47 L36 L39 L38 | L37 L35 L89 L38 | L89 L39 L50 L47 L42 L49 L38 | L62 L54 L56 L58 L66 L65 L60 | L60 L55 L66 L69 L58 L53 L54 | L58 L69 L63 L62 | L70 L87 L73 L85 L72 L75 L74 | L73 L71 L80 L74 | L80 L75 L83 L85 L87 L76 L74